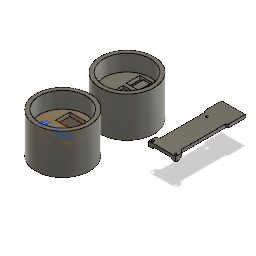
tstick_cap v71(Fusion360) (Autodesk Fusion 360 design; units mm, degrees)
Autodesk Fusion 360 part; units mm, degrees
sketch "Sketch1" plane through (0, 0, 0) normal (0, 1, 0) x (1, 0, 0) in component "battery_cap"
  circle A0 centre (0, 0) radius 21.25
  circle A1 centre (0, 0) radius 24.75
  dimension "d29" = 42.5
  dimension "d30" = 3.5
  constraint coincident A0.centre A1.centre
  measures "d29" diameter of A0
extrude "Extrude4" add sketch "Sketch1" against normal blind 3.5 contours A0 | A1 makes body 1 in component "battery_cap"
extrude "Extrude5" add sketch "Sketch1" along normal blind 15 bodies 1 in component "battery_cap"
sketch "Sketch2" plane through (0, -3.5, 0) normal (0, -1, 0) x (1, 0, 0) in component "battery_cap"
  circle A0 centre (0, 0) radius 24.75
  circle A1 centre (0, 0) radius 21.25
extrude "Extrude6" add sketch "Sketch2" along normal blind 15 bodies 1 in component "battery_cap"
sketch "switch_battery" plane through (0, -3.5, 0) normal (0, -1, 0) x (1, 0, 0) in component "battery_cap"
  circle A0 centre (0, 0) radius 21.25
  line L0 (0, 0) -> (0, 32) construction
  line L1 (0, 0) -> (28, 0) construction
  line L2 (28, 0) -> (27, 0)
  line L3 (9.5, -16) -> (-9.5, -16)
  line L4 (-9.5, -16) -> (-9.5, -3)
  line L5 (-9.5, -3) -> (9.5, -3)
  line L6 (9.5, -3) -> (9.5, -16)
  line L7 (9.5, -16) -> (-9.5, -3) construction
  line L8 (-9.5, -16) -> (9.5, -3) construction
  line L9 (11.725, 6.6) -> (-11.725, 6.6)
  line L10 (-11.725, 6.6) -> (-11.725, 1)
  line L11 (-11.725, 1) -> (11.725, 1)
  line L12 (11.725, 1) -> (11.725, 6.6)
  line L13 (11.725, 6.6) -> (-11.725, 1) construction
  line L14 (-11.725, 6.6) -> (11.725, 1) construction
  line L15 (11.725, 6.6) -> (11.725, 8.6)
  line L16 (-11.725, 6.6) -> (-11.725, 8.6)
  line L17 (-11.725, 8.6) -> (11.725, 8.6)
  line L18 (11.725, 1) -> (11.725, -1)
  line L19 (-11.725, 1) -> (-11.725, -1)
  line L20 (-11.725, -1) -> (11.725, -1)
  point P0 (0, -9.5)
  point P1 (0, 3.8)
  dimension "d48" = 19
  dimension "d49" = 13
  dimension "d50" = 3
  dimension "d51" = 23.45
  dimension "d52" = 5.6
  dimension "d53" = 1
  dimension "d181" = 2
  dimension "d182" = 2
  constraint coincident A0.centre L0.start
  constraint vertical L0
  constraint perpendicular L0 L1
  constraint coincident L1 L2.end
  constraint perpendicular L3 L4
  constraint parallel L3 L5
  constraint parallel L4 L6
  constraint horizontal L3
  constraint coincident L7 P0
  constraint coincident L8 P0
  constraint coincident L0 P0
  constraint perpendicular L9 L10
  constraint parallel L9 L11
  constraint parallel L10 L12
  constraint horizontal L9
  constraint coincident L13 P1
  constraint coincident L14 P1
  constraint coincident L0 P1
  constraint perpendicular L9 L15
  constraint perpendicular L9 L16
  constraint perpendicular L15 L17
  constraint perpendicular L1 L18
  constraint perpendicular L11 L19
  constraint perpendicular L18 L20
  measures "d48" distance of L4.end L5.end
  measures "d49" distance of L3.end L4.end
  measures "d50" distance of A0.centre L5
  measures "d51" distance of L10.end L11.end
  measures "d52" distance of L9.end L10.end
  measures "d53" distance of A0.centre L11
  measures "d181" distance of L9 L17
  measures "d182" distance of L11 L20
extrude "Extrude13" add sketch "switch_battery" along normal blind 15 contours L9 L15 L16 L17 | L11 L18 L19 L20 bodies 1 in component "battery_cap"
extrude "Extrude7" cut sketch "switch_battery" against normal up to surface (3.5 mm away) contours L3 L4 L5 L6 bodies 1 in component "battery_cap"
sketch "Sketch1 (2)" plane through (0, 0, 0) normal (0, 1, 0) x (1, 0, 0) in component "esp_cap"
  circle A0 centre (0, 0) radius 21.25
  circle A1 centre (0, 0) radius 24.75
  dimension "d29_1" = 42.5
  dimension "d30_1" = 3.5
  constraint coincident A0.centre A1.centre
  measures "d29_1" diameter of A0
extrude "Extrude4'" add sketch "Sketch1 (2)" against normal blind 3.5 separate body contours A0 | A1 makes body 2 in component "esp_cap"
extrude "Extrude5'" add sketch "Sketch1 (2)" along normal blind 15 bodies 2 in component "esp_cap"
sketch "Sketch2 (2)" plane through (0, -3.5, 0) normal (0, -1, 0) x (1, 0, 0) in component "esp_cap"
  circle A0 centre (0, 0) radius 24.75
  circle A1 centre (0, 0) radius 21.25
extrude "Extrude6'" add sketch "Sketch2 (2)" along normal blind 18.5 bodies 2 in component "esp_cap"
sketch "botton" plane through (0, -3.5, 0) normal (0, -1, 0) x (1, 0, 0) in component "esp_cap"
  circle A0 centre (0, 0) radius 21.25
  line L0 (0, 0) -> (0, 32) construction
  line L1 (0, 0) -> (30, 0) construction
  line L2 (-12.5, 6.5) -> (12.5, 6.5)
  line L3 (12.5, 6.5) -> (12.5, 5)
  line L4 (12.5, 5) -> (-12.5, 5)
  line L5 (-12.5, 5) -> (-12.5, 6.5)
  line L6 (-12.5, 6.5) -> (12.5, 5) construction
  line L7 (12.5, 6.5) -> (-12.5, 5) construction
  line L8 (7.4, 4.9) -> (12.4, 4.9)
  line L9 (12.4, 4.9) -> (12.4, -2.1)
  line L10 (12.4, -2.1) -> (7.4, -2.1)
  line L11 (7.4, -2.1) -> (7.4, 4.9)
  line L12 (7.4, 4.9) -> (12.4, -2.1) construction
  line L13 (12.4, 4.9) -> (7.4, -2.1) construction
  line L14 (-3.5, 4.9) -> (6.5, 4.9)
  line L15 (6.5, 4.9) -> (6.5, -0.1)
  line L16 (6.5, -0.1) -> (-3.5, -0.1)
  line L17 (-3.5, -0.1) -> (-3.5, 4.9)
  line L18 (-3.5, 4.9) -> (6.5, -0.1) construction
  line L19 (6.5, 4.9) -> (-3.5, -0.1) construction
  line L20 (0, 0) -> (0, -28) construction
  circle A1 centre (0, -12) radius 4
  line L21 (-6.25, -5.75) -> (6.25, -5.75)
  line L22 (6.25, -5.75) -> (6.25, -18.25)
  line L23 (6.25, -18.25) -> (-6.25, -18.25)
  line L24 (-6.25, -18.25) -> (-6.25, -5.75)
  line L25 (-6.25, -5.75) -> (6.25, -18.25) construction
  line L26 (6.25, -5.75) -> (-6.25, -18.25) construction
  line L27 (0, -12) -> (-10.4008, -12) construction
  line L28 (0, -12) -> (10, -12) construction
  line L29 (7.25, -13.5) -> (6.25, -13.5)
  line L30 (6.25, -13.5) -> (6.25, -10.5)
  line L31 (6.25, -10.5) -> (7.25, -10.5)
  line L32 (7.25, -10.5) -> (7.25, -13.5)
  line L33 (7.25, -13.5) -> (6.25, -10.5) construction
  line L34 (6.25, -13.5) -> (7.25, -10.5) construction
  line L35 (-7.25, -13.5) -> (-6.25, -13.5)
  line L36 (-6.25, -10.5) -> (-7.25, -10.5)
  line L37 (-7.25, -10.5) -> (-7.25, -13.5)
  line L38 (-6.25, -13.5) -> (-6.25, -10.5)
  line L39 (7.5, 5) -> (7.5, 6.5)
  line L40 (-7.5, 5) -> (-7.5, 6.5)
  line L41 (12.5, 6.5) -> (7.5, 6.5)
  line L42 (7.5, 9.75) -> (12.5, 9.75)
  line L43 (12.5, 9.75) -> (12.5, 6.5)
  line L44 (-12.5, 6.5) -> (-7.5, 6.5)
  line L45 (-7.1372, 9.75) -> (-12.5, 9.75)
  line L46 (-12.5, 9.75) -> (-12.5, 6.5)
  line L47 (12.5, 9.75) -> (-12.5, 9.75)
  line L48 (-12.5, 9.75) -> (-12.5, 11.25)
  line L49 (-12.5, 11.25) -> (12.5, 11.25)
  line L50 (12.5, 11.25) -> (12.5, 9.75)
  line L51 (11, 6.5) -> (11, 11.5)
  line L52 (-11, 6.5) -> (-11, 9.75)
  point P0 (0, 5.75)
  point P1 (9.9, 1.4)
  point P2 (1.5, 2.4)
  point P3 (0, -12)
  point P4 (6.75, -12)
  dimension "d65" = 25
  dimension "d66" = 1.5
  dimension "d67" = 5
  dimension "d70" = 5
  dimension "d71" = 7
  dimension "d72" = 0.1
  dimension "d74" = 10
  dimension "d75" = 5
  dimension "d76" = 0.1
  dimension "d82" = 0.1
  dimension "d83" = 9
  dimension "d111" = 8
  dimension "d112" = 12
  dimension "d113" = 12.5
  dimension "d114" = 12.5
  dimension "d117" = 1
  dimension "d118" = 3
  dimension "d119" = 6.25
  dimension "d200" = 5
  dimension "d201" = 5
  dimension "d202" = 3.25
  dimension "d203" = 3.25
  dimension "d204" = 1.5
  dimension "d205" = 1.5
  dimension "d206" = 1.5
  constraint coincident A0.centre L0.start
  constraint vertical L0
  constraint perpendicular L0 L1
  constraint perpendicular L2 L3
  constraint parallel L2 L4
  constraint parallel L3 L5
  constraint horizontal L2
  constraint coincident L6 P0
  constraint coincident L7 P0
  constraint coincident L0 P0
  constraint perpendicular L8 L9
  constraint parallel L8 L10
  constraint parallel L9 L11
  constraint horizontal L8
  constraint coincident L12 P1
  constraint coincident L13 P1
  constraint perpendicular L14 L15
  constraint parallel L14 L16
  constraint parallel L15 L17
  constraint horizontal L14
  constraint coincident L18 P2
  constraint coincident L19 P2
  constraint parallel L0 L20
  constraint coincident L20 P3
  constraint perpendicular L21 L22
  constraint parallel L21 L23
  constraint parallel L22 L24
  constraint horizontal L21
  constraint coincident L25 P3
  constraint coincident L26 P3
  constraint coincident P3 A1.centre
  constraint horizontal L27
  constraint perpendicular L20 L28
  constraint perpendicular L29 L30
  constraint parallel L29 L31
  constraint parallel L30 L32
  constraint horizontal L29
  constraint coincident L33 P4
  constraint coincident L34 P4
  constraint coincident L28 P4
  constraint symmetric L20 L29.start L35.start
  constraint symmetric L20 L29.end L35.end
  constraint symmetric L20 L30.end L36.start
  constraint symmetric L20 L31.end L36.end
  constraint coincident L4 L39.start
  constraint coincident L2 L39.end
  constraint perpendicular L2 L39
  constraint coincident L4 L40.start
  constraint coincident L2 L40.end
  constraint perpendicular L2 L40
  constraint parallel L41 L42
  constraint parallel L44 L45
  constraint perpendicular L47 L48
  constraint parallel L47 L49
  constraint parallel L48 L50
  constraint vertical L51
  constraint coincident L41 L51.start
  constraint coincident L2 L52.start
  constraint coincident L47 L52.end
  constraint perpendicular L47 L52
  measures "d65" distance of L3.end L4.end
  measures "d66" distance of L2.end L3.end
  measures "d67" distance of A0.centre L4
  measures "d70" distance of L9 L11
  measures "d71" distance of L8 L10
  measures "d72" distance of L4 L8
  measures "d74" distance of L15.end L16.end
  measures "d75" distance of L14.end L15.end
  measures "d76" distance of L4 L14
  measures "d82" distance of L3 L9
  measures "d83" distance of L5 L17
  measures "d111" diameter of A1
  measures "d112" distance of A0.centre P3
  measures "d113" distance of L22.end L23.end
  measures "d114" distance of L21.end L22.end
  measures "d117" distance of L30.end L31.end
  measures "d118" distance of L29 L31
  measures "d119" distance of P3 L30
  measures "d200" distance of L3 L39
  measures "d201" distance of L5 L40
  measures "d202" distance of L44 L45
  measures "d203" distance of L2 L42
  measures "d204" distance of L47 L49
  measures "d205" distance of L43 L51
  measures "d206" distance of L46 L52
extrude "Extrude30" add sketch "botton" along normal blind 18.5 contours L2 L44 L45 L46 L47 L52 | L2 L4 L5 L40 L44 | L42 L45 L47 L48 L49 L51 | L2 L3 L4 L39 L41 | L42 L47 L49 L50 L51 | L2 L41 L42 L43 L47 L51 bodies 2 in component "esp_cap"
extrude "Extrude11" cut sketch "botton" against normal up to surface (3.5 mm away) contours L8 L9 L10 L11 bodies 2 in component "esp_cap"
extrude "Extrude12" cut sketch "botton" against normal up to surface (3.5 mm away) contours L14 L15 L16 L17 bodies 2 in component "esp_cap"
sketch "top" plane through (0, 0, 0) normal (0, 1, 0) x (-1, 0, 0) in component "esp_cap"
  line L0 (3.5, 4.9) -> (3.5, -0.1)
  line L1 (3.5, -0.1) -> (-6.5, -0.1)
  line L2 (-6.5, 4.9) -> (3.5, 4.9)
  line L3 (-7.4, 4.9) -> (-7.4, -2.1)
  line L4 (-7.4, -2.1) -> (-12.4, -2.1)
  line L5 (-12.4, -2.1) -> (-12.4, 4.9)
  circle A0 centre (0, 0) radius 21.25
  line L6 (0, 0) -> (-32, 0) construction
  line L7 (0, 0) -> (0, -28) construction
  line L8 (-9, 7.4) -> (6, 7.4)
  line L9 (6, 7.4) -> (6, -2.6)
  line L10 (6, -2.6) -> (-9, -2.6)
  line L11 (-9, -2.6) -> (-9, 7.4)
  line L12 (-6.5, -0.1) -> (-6.5, 4.9)
  line L13 (-12.4, 4.9) -> (-7.4, 4.9)
  line L14 (0, 0) -> (27, 0) construction
  line L15 (-6, -5.7474) -> (6.5, -5.7474)
  line L16 (6.5, -5.7474) -> (6.5, -18.2474)
  line L17 (6.5, -18.2474) -> (-6, -18.2474)
  line L18 (-6, -18.2474) -> (-6, -5.7474)
  line L19 (-6, -5.7474) -> (6.5, -18.2474) construction
  line L20 (6.5, -5.7474) -> (-6, -18.2474) construction
  line L21 (3.375, -18.2474) -> (-2.875, -18.2474)
  line L22 (-2.875, -18.2474) -> (-2.875, -5.7474)
  line L23 (-2.875, -5.7474) -> (3.375, -5.7474)
  line L24 (3.375, -5.7474) -> (3.375, -18.2474)
  line L25 (3.375, -18.2474) -> (-2.875, -5.7474) construction
  line L26 (-2.875, -18.2474) -> (3.375, -5.7474) construction
  line L27 (10.5318, 13.8673) -> (10.5318, 8.8166)
  line L28 (10.5318, 8.8166) -> (12.4185, 8.8166)
  line L29 (12.4185, 8.8166) -> (12.4185, 8.1408)
  line L30 (12.4185, 8.1408) -> (7.8794, 8.1408)
  line L31 (7.8794, 8.1408) -> (7.8794, 8.8166)
  line L32 (7.8794, 8.8166) -> (9.7739, 8.8166)
  line L33 (9.7739, 8.8166) -> (9.7739, 13.8673)
  line L34 (9.7739, 13.8673) -> (10.5318, 13.8673)
  line L35 (7.4653, 12.1486) -> (7.4653, 11.4416)
  line L36 (7.4653, 11.4416) -> (5.3052, 11.4416)
  line L37 (5.3052, 11.4416) -> (5.3052, 12.1486)
  line L38 (5.3052, 12.1486) -> (7.4653, 12.1486)
  line L39 (4.6958, 12.0275) -> (3.981, 11.965)
  spline S0 degree 3 poles (3.981, 11.965) (3.9608, 12.0982) (3.9232, 12.3477) (3.8027, 12.5689) (3.7466, 12.672) knots 0 0 0 0 0.040051 0.074995 0.074995 0.074995 0.074995
  spline S1 degree 3 poles (3.7466, 12.672) (3.6718, 12.7606) (3.5115, 12.9503) (3.2878, 13.0592) (3.1685, 13.1173) knots 0 0 0 0 0.034396 0.07369 0.07369 0.07369 0.07369
  spline S2 degree 3 poles (3.1685, 13.1173) (3.0315, 13.1663) (2.7474, 13.2679) (2.4458, 13.2794) (2.2896, 13.2853) knots 0 0 0 0 0.043374 0.08995 0.08995 0.08995 0.08995
  spline S3 degree 3 poles (2.2896, 13.2853) (2.1524, 13.2811) (1.8911, 13.2731) (1.6422, 13.194) (1.5239, 13.1564) knots 0 0 0 0 0.040947 0.077974 0.077974 0.077974 0.077974
  spline S4 degree 3 poles (1.5239, 13.1564) (1.4226, 13.1124) (1.2331, 13.0302) (1.0957, 12.8764) (1.0318, 12.8048) knots 0 0 0 0 0.032675 0.061126 0.061126 0.061126 0.061126
  spline S5 degree 3 poles (1.0318, 12.8048) (0.9839, 12.7283) (0.8895, 12.5774) (0.8749, 12.4001) (0.8677, 12.3127) knots 0 0 0 0 0.026644 0.052557 0.052557 0.052557 0.052557
  spline S6 degree 3 poles (0.8677, 12.3127) (0.8737, 12.2263) (0.8857, 12.0566) (0.9784, 11.914) (1.0239, 11.8439) knots 0 0 0 0 0.025496 0.050141 0.050141 0.050141 0.050141
  spline S7 degree 3 poles (1.0239, 11.8439) (1.0898, 11.7771) (1.237, 11.6276) (1.4319, 11.548) (1.5396, 11.5041) knots 0 0 0 0 0.027866 0.062324 0.062324 0.062324 0.062324
  spline S8 degree 3 poles (1.5396, 11.5041) (1.6626, 11.4648) (1.9983, 11.3575) (2.3416, 11.2774) (2.5591, 11.2267) knots 0 0 0 0 0.038735 0.105693 0.105693 0.105693 0.105693
  spline S9 degree 3 poles (2.5591, 11.2267) (2.7852, 11.1721) (3.1633, 11.0809) (3.5208, 10.9286) (3.6646, 10.8673) knots 0 0 0 0 0.069608 0.116413 0.116413 0.116413 0.116413
  spline S10 degree 3 poles (3.6646, 10.8673) (3.7905, 10.7947) (4.0295, 10.6569) (4.1981, 10.4391) (4.2778, 10.3361) knots 0 0 0 0 0.043147 0.081832 0.081832 0.081832 0.081832
  spline S11 degree 3 poles (4.2778, 10.3361) (4.336, 10.2255) (4.4536, 10.0015) (4.4692, 9.749) (4.4771, 9.6212) knots 0 0 0 0 0.037035 0.074961 0.074961 0.074961 0.074961
  spline S12 degree 3 poles (4.4771, 9.6212) (4.4664, 9.4786) (4.445, 9.1907) (4.3027, 8.9394) (4.231, 8.8127) knots 0 0 0 0 0.042344 0.085459 0.085459 0.085459 0.085459
  spline S13 degree 3 poles (4.231, 8.8127) (4.137, 8.693) (3.9427, 8.4455) (3.6589, 8.309) (3.5122, 8.2384) knots 0 0 0 0 0.045005 0.093093 0.093093 0.093093 0.093093
  spline S14 degree 3 poles (3.5122, 8.2384) (3.3474, 8.1815) (3.0071, 8.0639) (2.6471, 8.0502) (2.4614, 8.0431) knots 0 0 0 0 0.052008 0.107399 0.107399 0.107399 0.107399
  spline S15 degree 3 poles (2.4614, 8.0431) (2.2599, 8.0499) (1.8756, 8.0629) (1.5129, 8.1898) (1.3403, 8.2502) knots 0 0 0 0 0.060087 0.114591 0.114591 0.114591 0.114591
  spline S16 degree 3 poles (1.3403, 8.2502) (1.1883, 8.3241) (0.8925, 8.4679) (0.6892, 8.7262) (0.5903, 8.8517) knots 0 0 0 0 0.049979 0.097264 0.097264 0.097264 0.097264
  spline S17 degree 3 poles (0.5903, 8.8517) (0.5132, 8.9901) (0.3564, 9.2712) (0.325, 9.5915) (0.3091, 9.7541) knots 0 0 0 0 0.047003 0.095424 0.095424 0.095424 0.095424
  line L40 (0.3091, 9.7541) -> (1.0357, 9.8087)
  spline S18 degree 3 poles (1.0357, 9.8087) (1.0631, 9.6421) (1.1148, 9.328) (1.3321, 9.0969) (1.4341, 8.9884) knots 0 0 0 0 0.049369 0.093051 0.093051 0.093051 0.093051
  spline S19 degree 3 poles (1.4341, 8.9884) (1.5697, 8.9078) (1.8751, 8.7263) (2.2319, 8.7165) (2.4302, 8.7111) knots 0 0 0 0 0.046599 0.104923 0.104923 0.104923 0.104923
  spline S20 degree 3 poles (2.4302, 8.7111) (2.6334, 8.7143) (2.99, 8.72) (3.3005, 8.8913) (3.4341, 8.965) knots 0 0 0 0 0.05981 0.104943 0.104943 0.104943 0.104943
  spline S21 degree 3 poles (3.4341, 8.965) (3.5252, 9.0506) (3.7014, 9.216) (3.7319, 9.455) (3.7466, 9.5705) knots 0 0 0 0 0.036237 0.070062 0.070062 0.070062 0.070062
  spline S22 degree 3 poles (3.7466, 9.5705) (3.7377, 9.6685) (3.72, 9.8627) (3.5889, 10.0069) (3.5239, 10.0783) knots 0 0 0 0 0.028671 0.056816 0.056816 0.056816 0.056816
  spline S23 degree 3 poles (3.5239, 10.0783) (3.3944, 10.1507) (3.0385, 10.3497) (2.638, 10.4345) (2.3833, 10.4884) knots 0 0 0 0 0.04433 0.121785 0.121785 0.121785 0.121785
  spline S24 degree 3 poles (2.3833, 10.4884) (2.1212, 10.5463) (1.6903, 10.6414) (1.276, 10.7925) (1.1138, 10.8517) knots 0 0 0 0 0.080411 0.132172 0.132172 0.132172 0.132172
  spline S25 degree 3 poles (1.1138, 10.8517) (0.9611, 10.9293) (0.6748, 11.0749) (0.4708, 11.3222) (0.3755, 11.4377) knots 0 0 0 0 0.050729 0.095154 0.095154 0.095154 0.095154
  spline S26 degree 3 poles (0.3755, 11.4377) (0.306, 11.561) (0.1639, 11.8132) (0.1463, 12.1024) (0.1372, 12.2502) knots 0 0 0 0 0.041894 0.08566 0.08566 0.08566 0.08566
  spline S27 degree 3 poles (0.1372, 12.2502) (0.1488, 12.4014) (0.1722, 12.7083) (0.3226, 12.9771) (0.3989, 13.1134) knots 0 0 0 0 0.044913 0.091178 0.091178 0.091178 0.091178
  spline S28 degree 3 poles (0.3989, 13.1134) (0.4983, 13.2414) (0.7035, 13.5057) (0.9999, 13.6618) (1.1528, 13.7423) knots 0 0 0 0 0.048003 0.099191 0.099191 0.099191 0.099191
  spline S29 degree 3 poles (1.1528, 13.7423) (1.3241, 13.8073) (1.6789, 13.9417) (2.0582, 13.9571) (2.2544, 13.965) knots 0 0 0 0 0.054571 0.11304 0.11304 0.11304 0.11304
  spline S30 degree 3 poles (2.2544, 13.965) (2.495, 13.9589) (2.9416, 13.9475) (3.3642, 13.8044) (3.5591, 13.7384) knots 0 0 0 0 0.071708 0.133092 0.133092 0.133092 0.133092
  spline S31 degree 3 poles (3.5591, 13.7384) (3.7236, 13.6545) (4.0486, 13.4886) (4.2727, 13.2008) (4.3833, 13.0587) knots 0 0 0 0 0.054682 0.107998 0.107998 0.107998 0.107998
  spline S32 degree 3 poles (4.3833, 13.0587) (4.4706, 12.9002) (4.6476, 12.5787) (4.6796, 12.2129) (4.6958, 12.0275) knots 0 0 0 0 0.053651 0.108817 0.108817 0.108817 0.108817
  line L41 (-2.3432, 13.2384) -> (-2.4448, 13.8595)
  spline S33 degree 3 poles (-2.4448, 13.8595) (-2.3514, 13.8777) (-2.1758, 13.9119) (-1.9971, 13.9188) (-1.9136, 13.922) knots 0 0 0 0 0.028513 0.053562 0.053562 0.053562 0.053562
  spline S34 degree 3 poles (-1.9136, 13.922) (-1.7985, 13.9198) (-1.5926, 13.9159) (-1.4034, 13.8361) (-1.3198, 13.8009) knots 0 0 0 0 0.034119 0.061085 0.061085 0.061085 0.061085
  spline S35 degree 3 poles (-1.3198, 13.8009) (-1.2553, 13.7587) (-1.1306, 13.6771) (-1.058, 13.5472) (-1.0229, 13.4845) knots 0 0 0 0 0.022757 0.043965 0.043965 0.043965 0.043965
  spline S36 degree 3 poles (-1.0229, 13.4845) (-0.9982, 13.3824) (-0.9323, 13.1097) (-0.9352, 12.8284) (-0.937, 12.6525) knots 0 0 0 0 0.03143 0.083915 0.083915 0.083915 0.083915
  line L42 (-0.937, 12.6525) -> (-0.937, 10.2658)
  line L43 (-0.937, 10.2658) -> (-0.4214, 10.2658)
  line L44 (-0.4214, 10.2658) -> (-0.4214, 9.7189)
  line L45 (-0.4214, 9.7189) -> (-0.937, 9.7189)
  line L46 (-0.937, 9.7189) -> (-0.937, 8.6916)
  line L47 (-0.937, 8.6916) -> (-1.6362, 8.2697)
  line L48 (-1.6362, 8.2697) -> (-1.6362, 9.7189)
  line L49 (-1.6362, 9.7189) -> (-2.3432, 9.7189)
  line L50 (-2.3432, 9.7189) -> (-2.3432, 10.2658)
  line L51 (-2.3432, 10.2658) -> (-1.6362, 10.2658)
  line L52 (-1.6362, 10.2658) -> (-1.6362, 12.6916)
  spline S37 degree 3 poles (-1.6362, 12.6916) (-1.6352, 12.7744) (-1.6337, 12.9047) (-1.6613, 13.0319) (-1.6714, 13.0783) knots 0 0 0 0 0.024723 0.038934 0.038934 0.038934 0.038934
  spline S38 degree 3 poles (-1.6714, 13.0783) (-1.6863, 13.1055) (-1.7162, 13.1603) (-1.7669, 13.1967) (-1.7925, 13.215) knots 0 0 0 0 0.009183 0.018473 0.018473 0.018473 0.018473
  spline S39 degree 3 poles (-1.7925, 13.215) (-1.8265, 13.2298) (-1.9035, 13.2632) (-1.9877, 13.2648) (-2.0347, 13.2658) knots 0 0 0 0 0.01103 0.024955 0.024955 0.024955 0.024955
  spline S40 degree 3 poles (-2.0347, 13.2658) (-2.08, 13.2642) (-2.1833, 13.2605) (-2.2857, 13.2464) (-2.3432, 13.2384) knots 0 0 0 0 0.013591 0.030998 0.030998 0.030998 0.030998
  line L53 (-3.0347, 8.9494) -> (-3.0347, 8.1408)
  line L54 (-3.0347, 8.1408) -> (-3.7378, 8.1408)
  line L55 (-3.7378, 8.1408) -> (-3.7378, 8.9494)
  line L56 (-3.7378, 8.9494) -> (-3.0347, 8.9494)
  line L57 (-3.0347, 13.8673) -> (-3.0347, 9.7189)
  line L58 (-3.0347, 9.7189) -> (-3.7378, 9.7189)
  line L59 (-3.7378, 9.7189) -> (-3.7378, 13.8673)
  line L60 (-3.7378, 13.8673) -> (-3.0347, 13.8673)
  line L61 (-7.5151, 12.3478) -> (-8.2065, 12.4377)
  spline S41 degree 3 poles (-8.2065, 12.4377) (-8.1575, 12.6599) (-8.0634, 13.0865) (-7.7666, 13.4058) (-7.6245, 13.5588) knots 0 0 0 0 0.066897 0.128377 0.128377 0.128377 0.128377
  spline S42 degree 3 poles (-7.6245, 13.5588) (-7.4576, 13.6761) (-7.1144, 13.9174) (-6.6953, 13.9463) (-6.48, 13.9611) knots 0 0 0 0 0.059996 0.123397 0.123397 0.123397 0.123397
  spline S43 degree 3 poles (-6.48, 13.9611) (-6.2129, 13.9411) (-5.6956, 13.9024) (-5.3002, 13.5681) (-5.1089, 13.4064) knots 0 0 0 0 0.078096 0.151317 0.151317 0.151317 0.151317
  spline S44 degree 3 poles (-5.1089, 13.4064) (-4.9588, 13.1874) (-4.6304, 12.7082) (-4.6063, 12.1253) (-4.5932, 11.8087) knots 0 0 0 0 0.078115 0.17091 0.17091 0.17091 0.17091
  spline S45 degree 3 poles (-4.5932, 11.8087) (-4.6005, 11.5966) (-4.6142, 11.1929) (-4.751, 10.8131) (-4.8159, 10.633) knots 0 0 0 0 0.063234 0.120321 0.120321 0.120321 0.120321
  spline S46 degree 3 poles (-4.8159, 10.633) (-4.8984, 10.4763) (-5.0607, 10.1682) (-5.3496, 9.9744) (-5.4917, 9.8791) knots 0 0 0 0 0.052205 0.102672 0.102672 0.102672 0.102672
  spline S47 degree 3 poles (-5.4917, 9.8791) (-5.6478, 9.805) (-5.962, 9.656) (-6.3092, 9.6355) (-6.4839, 9.6252) knots 0 0 0 0 0.05132 0.103272 0.103272 0.103272 0.103272
  spline S48 degree 3 poles (-6.4839, 9.6252) (-6.6943, 9.636) (-7.0931, 9.6566) (-7.4302, 9.8687) (-7.5893, 9.9689) knots 0 0 0 0 0.062024 0.1175 0.1175 0.1175 0.1175
  spline S49 degree 3 poles (-7.5893, 9.9689) (-7.7205, 10.0984) (-7.9944, 10.369) (-8.0902, 10.7428) (-8.1401, 10.9377) knots 0 0 0 0 0.054233 0.113322 0.113322 0.113322 0.113322
  line L62 (-8.1401, 10.9377) -> (-7.4565, 11.0431)
  spline S50 degree 3 poles (-7.4565, 11.0431) (-7.4211, 10.9155) (-7.355, 10.6776) (-7.1868, 10.4976) (-7.1089, 10.4142) knots 0 0 0 0 0.039056 0.072807 0.072807 0.072807 0.072807
  spline S51 degree 3 poles (-7.1089, 10.4142) (-7.0212, 10.3527) (-6.8418, 10.2269) (-6.623, 10.2113) (-6.5112, 10.2033) knots 0 0 0 0 0.031506 0.06445 0.06445 0.06445 0.06445
  spline S52 degree 3 poles (-6.5112, 10.2033) (-6.3432, 10.2183) (-6.0117, 10.2481) (-5.7681, 10.4744) (-5.6479, 10.5861) knots 0 0 0 0 0.049087 0.09686 0.09686 0.09686 0.09686
  spline S53 degree 3 poles (-5.6479, 10.5861) (-5.5515, 10.7455) (-5.3293, 11.1128) (-5.3207, 11.5447) (-5.3159, 11.7892) knots 0 0 0 0 0.054986 0.126756 0.126756 0.126756 0.126756
  spline S54 degree 3 poles (-5.3159, 11.7892) (-5.32, 12.0363) (-5.3272, 12.4701) (-5.5432, 12.8434) (-5.6362, 13.0041) knots 0 0 0 0 0.072611 0.127467 0.127467 0.127467 0.127467
  spline S55 degree 3 poles (-5.6362, 13.0041) (-5.7521, 13.1146) (-5.9863, 13.3381) (-6.309, 13.3679) (-6.4722, 13.383) knots 0 0 0 0 0.046586 0.094217 0.094217 0.094217 0.094217
  spline S56 degree 3 poles (-6.4722, 13.383) (-6.6032, 13.3736) (-6.8584, 13.3552) (-7.0637, 13.2031) (-7.1636, 13.1291) knots 0 0 0 0 0.038515 0.075027 0.075027 0.075027 0.075027
  spline S57 degree 3 poles (-7.1636, 13.1291) (-7.2484, 13.026) (-7.4356, 12.7985) (-7.487, 12.5072) (-7.5151, 12.3478) knots 0 0 0 0 0.039394 0.086964 0.086964 0.086964 0.086964
  line L63 (-8.812, 13.8673) -> (-8.812, 8.1408)
  line L64 (-8.812, 8.1408) -> (-9.5151, 8.1408)
  line L65 (-9.5151, 8.1408) -> (-9.5151, 11.4064)
  line L66 (-9.5151, 11.4064) -> (-11.1792, 9.7189)
  line L67 (-11.1792, 9.7189) -> (-12.0893, 9.7189)
  line L68 (-12.0893, 9.7189) -> (-10.5034, 11.258)
  line L69 (-10.5034, 11.258) -> (-12.2495, 13.8673)
  line L70 (-12.2495, 13.8673) -> (-11.3823, 13.8673)
  line L71 (-11.3823, 13.8673) -> (-10.0112, 11.7462)
  line L72 (-10.0112, 11.7462) -> (-9.5151, 12.2228)
  line L73 (-9.5151, 12.2228) -> (-9.5151, 13.8673)
  line L74 (-9.5151, 13.8673) -> (-8.812, 13.8673)
  line L75 (7.6067, 18.9989) -> (7.6067, 14.704)
  line L76 (7.6067, 14.704) -> (7.0383, 14.704)
  line L77 (7.0383, 14.704) -> (7.0383, 18.9989)
  line L78 (7.0383, 18.9989) -> (7.6067, 18.9989)
  line L79 (6.0363, 18.9989) -> (6.0363, 14.704)
  line L80 (6.0363, 14.704) -> (4.5568, 14.704)
  spline S58 degree 3 poles (4.5568, 14.704) (4.4092, 14.7046) (4.1526, 14.7056) (3.8996, 14.7477) (3.7922, 14.7655) knots 0 0 0 0 0.044192 0.07682 0.07682 0.07682 0.07682
  spline S59 degree 3 poles (3.7922, 14.7655) (3.6749, 14.7985) (3.4461, 14.863) (3.2553, 15.0043) (3.1623, 15.0731) knots 0 0 0 0 0.036228 0.07062 0.07062 0.07062 0.07062
  spline S60 degree 3 poles (3.1623, 15.0731) (3.0557, 15.1769) (2.8384, 15.3885) (2.7172, 15.6667) (2.6555, 15.8085) knots 0 0 0 0 0.044179 0.090072 0.090072 0.090072 0.090072
  spline S61 degree 3 poles (2.6555, 15.8085) (2.6059, 15.9664) (2.5019, 16.2982) (2.4912, 16.6459) (2.4856, 16.828) knots 0 0 0 0 0.049425 0.103791 0.103791 0.103791 0.103791
  spline S62 degree 3 poles (2.4856, 16.828) (2.4892, 16.9826) (2.4961, 17.2759) (2.5665, 17.5606) (2.5998, 17.6952) knots 0 0 0 0 0.046231 0.087702 0.087702 0.087702 0.087702
  spline S63 degree 3 poles (2.5998, 17.6952) (2.6384, 17.8127) (2.711, 18.0336) (2.8348, 18.2302) (2.8928, 18.3221) knots 0 0 0 0 0.036947 0.069434 0.069434 0.069434 0.069434
  spline S64 degree 3 poles (2.8928, 18.3221) (2.9522, 18.3988) (3.0661, 18.5458) (3.2144, 18.658) (3.2854, 18.7118) knots 0 0 0 0 0.028941 0.055527 0.055527 0.055527 0.055527
  spline S65 degree 3 poles (3.2854, 18.7118) (3.3618, 18.7564) (3.5231, 18.8505) (3.7033, 18.8998) (3.7981, 18.9257) knots 0 0 0 0 0.026441 0.055764 0.055764 0.055764 0.055764
  spline S66 degree 3 poles (3.7981, 18.9257) (3.9049, 18.947) (4.1321, 18.9924) (4.3638, 18.9966) (4.4865, 18.9989) knots 0 0 0 0 0.032619 0.069359 0.069359 0.069359 0.069359
  line L81 (4.4865, 18.9989) -> (6.0363, 18.9989)
  line L82 (5.468, 18.4921) -> (4.551, 18.4921)
  spline S67 degree 3 poles (4.551, 18.4921) (4.4241, 18.4908) (4.1993, 18.4887) (3.981, 18.4359) (3.8859, 18.413) knots 0 0 0 0 0.037918 0.067164 0.067164 0.067164 0.067164
  spline S68 degree 3 poles (3.8859, 18.413) (3.8107, 18.3855) (3.6687, 18.3337) (3.5534, 18.2361) (3.4992, 18.1903) knots 0 0 0 0 0.023813 0.044936 0.044936 0.044936 0.044936
  spline S69 degree 3 poles (3.4992, 18.1903) (3.4347, 18.1142) (3.2977, 17.9527) (3.2245, 17.7536) (3.1858, 17.6483) knots 0 0 0 0 0.029693 0.063046 0.063046 0.063046 0.063046
  spline S70 degree 3 poles (3.1858, 17.6483) (3.1525, 17.5228) (3.0805, 17.2513) (3.0746, 16.9703) (3.0715, 16.8192) knots 0 0 0 0 0.038824 0.083958 0.083958 0.083958 0.083958
  spline S71 degree 3 poles (3.0715, 16.8192) (3.0754, 16.6173) (3.0823, 16.2569) (3.2294, 15.9292) (3.2942, 15.785) knots 0 0 0 0 0.059806 0.106748 0.106748 0.106748 0.106748
  spline S72 degree 3 poles (3.2942, 15.785) (3.3679, 15.6754) (3.5069, 15.4687) (3.7269, 15.353) (3.8303, 15.2987) knots 0 0 0 0 0.038914 0.0734 0.0734 0.0734 0.0734
  spline S73 degree 3 poles (3.8303, 15.2987) (3.9292, 15.2733) (4.1699, 15.2113) (4.4189, 15.211) (4.5656, 15.2108) knots 0 0 0 0 0.03053 0.07431 0.07431 0.07431 0.07431
  line L83 (4.5656, 15.2108) -> (5.468, 15.2108)
  line L84 (5.468, 15.2108) -> (5.468, 18.4921)
  line L85 (1.7209, 18.9989) -> (1.7209, 14.704)
  line L86 (1.7209, 14.704) -> (0.8654, 14.704)
  line L87 (0.8654, 14.704) -> (-0.1512, 17.745)
  spline S74 degree 3 poles (-0.1512, 17.745) (-0.1921, 17.8686) (-0.262, 18.0801) (-0.3286, 18.2925) (-0.3562, 18.3807) knots 0 0 0 0 0.039074 0.066801 0.066801 0.066801 0.066801
  spline S75 degree 3 poles (-0.3562, 18.3807) (-0.3872, 18.2842) (-0.4612, 18.054) (-0.5394, 17.8252) (-0.5848, 17.6923) knots 0 0 0 0 0.030412 0.072542 0.072542 0.072542 0.072542
  line L88 (-0.5848, 17.6923) -> (-1.6131, 14.704)
  line L89 (-1.6131, 14.704) -> (-2.3777, 14.704)
  line L90 (-2.3777, 14.704) -> (-2.3777, 18.9989)
  line L91 (-2.3777, 18.9989) -> (-1.8299, 18.9989)
  line L92 (-1.8299, 18.9989) -> (-1.8299, 15.4042)
  line L93 (-1.8299, 15.4042) -> (-0.5818, 18.9989)
  line L94 (-0.5818, 18.9989) -> (-0.0691, 18.9989)
  line L95 (-0.0691, 18.9989) -> (1.1731, 15.3426)
  line L96 (1.1731, 15.3426) -> (1.1731, 18.9989)
  line L97 (1.1731, 18.9989) -> (1.7209, 18.9989)
  line L98 (-3.3914, 18.9989) -> (-3.3914, 14.704)
  line L99 (-3.3914, 14.704) -> (-3.9598, 14.704)
  line L100 (-3.9598, 14.704) -> (-3.9598, 18.9989)
  line L101 (-3.9598, 18.9989) -> (-3.3914, 18.9989)
  line L102 (-4.9383, 18.9989) -> (-4.9383, 14.704)
  line L103 (-4.9383, 14.704) -> (-5.5066, 14.704)
  line L104 (-5.5066, 14.704) -> (-5.5066, 18.4921)
  line L105 (-5.5066, 18.4921) -> (-7.6219, 18.4921)
  line L106 (-7.6219, 18.4921) -> (-7.6219, 18.9989)
  line L107 (-7.6219, 18.9989) -> (-4.9383, 18.9989)
  point P0 (0.25, -11.9974)
  point P1 (0.25, -11.9974)
  point P2 (0.25, -11.9974)
  dimension "d149" = 2.5
  dimension "d150" = 2.5
  dimension "d151" = 2.5
  dimension "d153" = 2.5
  dimension "d155" = 12.5
  dimension "d156" = 12.5
  dimension "d158" = 12
  dimension "d159" = 6.25
  dimension "d160" = 12.5
  constraint coincident A0.centre L6.start
  constraint parallel L1 L6
  constraint perpendicular L6 L7
  constraint parallel L2 L8
  constraint parallel L0 L9
  constraint parallel L1 L10
  constraint perpendicular L9 L14
  constraint perpendicular L15 L16
  constraint parallel L15 L17
  constraint parallel L16 L18
  constraint horizontal L15
  constraint coincident L19 P2
  constraint coincident L20 P2
  constraint coincident P2 P1
  constraint perpendicular L21 L22
  constraint parallel L21 L23
  constraint parallel L22 L24
  constraint horizontal L21
  constraint coincident L25 P2
  constraint coincident L26 P2
  measures "d149" distance of L0 L9
  measures "d150" distance of L2 L8
  measures "d151" distance of L1 L10
  measures "d153" distance of L11 L12
  measures "d155" distance of L16.end L17.end
  measures "d156" distance of L15.end L16.end
  measures "d158" distance of A0.centre P2
  measures "d159" distance of L22.end L23.end
  measures "d160" distance of L21.end L22.end
extrude "Extrude14" cut sketch "top" against normal blind 1 contours L75 L76 L77 L78 | L79 L80 S58 S59 S60 S61 S62 S63 S64 S65 S66 L81 | L85 L86 L87 S74 S75 L88 L89 L90 L91 L92 L93 L94 L95 L96 L97 | L98 L99 L100 L101 | L102 L103 L104 L105 L106 L107 bodies 1 in component "battery_cap"
extrude "Extrude31" cut sketch "top" against normal blind 1 contours L75 L76 L77 L78 | L79 L80 S58 S59 S60 S61 S62 S63 S64 S65 S66 L81 | L85 L86 L87 S74 S75 L88 L89 L90 L91 L92 L93 L94 L95 L96 L97 | L98 L99 L100 L101 | L102 L103 L104 L105 L106 L107 bodies 2 in component "esp_cap"
extrude "Extrude27" add sketch "top" along normal blind 1 contours L27 L28 L29 L30 L31 L32 L33 L34 | L35 L36 L37 L38 | L39 S0 S1 S2 S3 S4 S5 S6 S7 S8 S9 S10 S11 S12 S13 S14 S15 S16 S17 L40 S18 S19 S20 S21 S22 S23 S24 S25 S26 S27 S28 S29 S30 S31 S32 | L41 S33 S34 S35 S36 L42 L43 L44 L45 L46 L47 L48 L49 L50 L51 L52 S37 S38 S39 S40 | L53 L54 L55 L56 | L57 L58 L59 L60 | L61 S41 S42 S43 S44 S45 S46 S47 S48 S49 L62 S50 S51 S52 S53 S54 S55 S56 S57 | L63 L64 L65 L66 L67 L68 L69 L70 L71 L72 L73 L74 bodies 2 in component "esp_cap"
extrude "Extrude17" cut sketch "top" against normal blind 2.5 contours L3 L4 L8 L9 L10 L11 L13 | L3 L4 L11 L13 bodies 2 in component "esp_cap"
extrude "Extrude24" cut sketch "top" against normal blind 2 contours L15 L17 L21 L22 L23 L24 bodies 2 in component "esp_cap"
extrude "Extrude25" cut sketch "top" against normal up to surface (3.5 mm away) contours L15 L17 L18 L22 | L15 L16 L17 L24 bodies 2 in component "esp_cap"
extrude "Extrude26" add 1 faces at (9, -0.8333, -2.4333) along direction (-1, 0, 0) up to surface (1.6 mm away) on bodies 2 bodies 2 in component "esp_cap"
move_face "OffsetFaces1" offset 3.5 1 faces at (23.4121, -18.5, -2.2853) on bodies 1 in component "battery_cap"
sketch "top (2)" plane through (0, 0, 0) normal (0, 1, 0) x (-1, 0, 0) in component "battery_cap"
  circle A0 centre (0, 0) radius 21.25
  line L0 (-9.5, -16) -> (-9.5, -3)
  line L1 (-9.5, -3) -> (9.5, -3)
  line L2 (9.5, -3) -> (9.5, -16)
  line L3 (9.5, -16) -> (-9.5, -16)
sketch "bed" plane through (0, 0, 0) normal (0, 1, 0) x (1, 0, 0) in component "esp_bed"
  line L0 (12.5, 32.75) -> (-12.5, 32.75)
  line L1 (-12.5, 32.75) -> (-12.5, -32.75)
  line L2 (-12.5, -32.75) -> (12.5, -32.75)
  line L3 (12.5, -32.75) -> (12.5, 32.75)
  line L4 (12.5, 32.75) -> (-12.5, -32.75) construction
  line L5 (-12.5, 32.75) -> (12.5, -32.75) construction
  circle A0 centre (10.5, -30.75) radius 1
  circle A1 centre (-10.5, -30.75) radius 1
  circle A2 centre (-5, 13.25) radius 1
  line L6 (10.5, -30.75) -> (10.5, 25) construction
  line L7 (-19, 17.75) -> (17, 17.75) construction
  line L8 (-12.5, 17.75) -> (-9.4847, 16.0091)
  line L9 (-9.4847, 16.0091) -> (-9.4847, -24.85)
  line L10 (-9.4847, -24.85) -> (-12.5, -27.3801)
  line L11 (-12.5, -27.3801) -> (-12.5, 17.75)
  line L12 (0, -32.75) -> (0, 40) construction
  line L13 (12.5, -27.3801) -> (12.5, 17.75)
  line L14 (9.4847, 16.0091) -> (9.4847, -24.85)
  line L15 (12.5, 17.75) -> (9.4847, 16.0091)
  line L16 (9.4847, -24.85) -> (12.5, -27.3801)
  line L17 (8.5, -28.75) -> (12.5, -28.75)
  line L18 (12.5, -28.75) -> (12.5, -32.75)
  line L19 (12.5, -32.75) -> (8.5, -32.75)
  line L20 (8.5, -32.75) -> (8.5, -28.75)
  line L21 (8.5, -28.75) -> (12.5, -32.75) construction
  line L22 (12.5, -28.75) -> (8.5, -32.75) construction
  line L23 (-8.5, -28.75) -> (-12.5, -28.75)
  line L24 (-12.5, -28.75) -> (-12.5, -32.75)
  line L25 (-12.5, -32.75) -> (-8.5, -32.75)
  line L26 (-8.5, -32.75) -> (-8.5, -28.75)
  line L27 (-8.5, -28.75) -> (-12.5, -32.75) construction
  line L28 (-12.5, -28.75) -> (-8.5, -32.75) construction
  line L29 (-3, 11.25) -> (-7, 11.25)
  line L30 (-7, 11.25) -> (-7, 15.25)
  line L31 (-7, 15.25) -> (-3, 15.25)
  line L32 (-3, 15.25) -> (-3, 11.25)
  line L33 (-3, 11.25) -> (-7, 15.25) construction
  line L34 (-7, 11.25) -> (-3, 15.25) construction
  line L35 (-10.5, -30.75) -> (-4, -30.75) construction
  line L36 (-9.4847, -24.85) -> (-9.4847, -31.5493) construction
  line L37 (11, 32.75) -> (-11, 32.75)
  line L38 (-11, 32.75) -> (-11, 17.75)
  line L39 (-11, 17.75) -> (11, 17.75)
  line L40 (11, 17.75) -> (11, 32.75)
  line L41 (11, 32.75) -> (-11, 17.75) construction
  line L42 (-11, 32.75) -> (11, 17.75) construction
  line L43 (11, 17.75) -> (12.5, 17.75)
  line L44 (-11, 17.75) -> (-12.5, 17.75)
  line L45 (11, 17.75) -> (11, 16.6229)
  line L46 (-11, 17.75) -> (-11, 16.6227)
  point P0 (10.5, -30.75)
  point P1 (-10.5, -30.75)
  point P2 (-5, 13.25)
  point P3 (0, 25.25)
  point P4 (0, 32.75)
  point P5 (0, 32.75)
  dimension "d185" = 65.5
  dimension "d186" = 25
  dimension "d189" = 2
  dimension "d190" = 2
  dimension "d191" = 2
  dimension "d192" = 2
  dimension "d193" = 2
  dimension "d194" = 2
  dimension "d195" = 2
  dimension "d197" = 44
  dimension "d209" = 15
  dimension "d211" = 60
  dimension "d212" = 50
  dimension "d213" = 4
  dimension "d214" = 4
  dimension "d215" = 4
  dimension "d216" = 4
  dimension "d221" = 4
  dimension "d222" = 4
  dimension "d224" = 5.9
  dimension "d227" = 15
  dimension "d229" = 7.5
  dimension "d230" = 22
  constraint perpendicular L0 L1
  constraint parallel L0 L2
  constraint parallel L1 L3
  constraint horizontal L0
  constraint coincident L4 origin
  constraint coincident L5 origin
  constraint coincident P0 A0.centre
  constraint parallel L3 L6
  constraint perpendicular L3 L7
  constraint coincident L7 L8.start
  constraint coincident L1 L8.start
  constraint coincident L4 L9.end
  constraint perpendicular L7 L9
  constraint coincident L1 L10.end
  constraint midpoint L2 L12.start
  constraint perpendicular L0 L12
  constraint symmetric L8.start L12 L13.end
  constraint symmetric L8.end L12 L14.start
  constraint symmetric L9.end L12 L14.end
  constraint symmetric L10.end L12 L13.start
  constraint perpendicular L17 L18
  constraint parallel L17 L19
  constraint parallel L18 L20
  constraint horizontal L17
  constraint coincident L21 P0
  constraint coincident L22 P0
  constraint perpendicular L23 L24
  constraint parallel L23 L25
  constraint parallel L24 L26
  constraint horizontal L23
  constraint coincident L27 P1
  constraint coincident L28 P1
  constraint coincident P1 A1.centre
  constraint perpendicular L29 L30
  constraint parallel L29 L31
  constraint parallel L30 L32
  constraint horizontal L29
  constraint coincident L33 P2
  constraint coincident L34 P2
  constraint coincident P2 A2.centre
  constraint perpendicular L26 L35
  constraint vertical L36
  constraint perpendicular L37 L38
  constraint parallel L37 L39
  constraint parallel L38 L40
  constraint horizontal L37
  constraint coincident L41 P3
  constraint coincident L42 P3
  constraint coincident L12 P3
  constraint midpoint L0 P5
  constraint midpoint L37 P5
  constraint perpendicular L13 L43
  constraint perpendicular L39 L45
  constraint vertical L46
  measures "d185" distance of L0.end L1.end
  measures "d186" distance of L1.end L2.end
  measures "d189" diameter of A0
  measures "d190" diameter of A1
  measures "d191" diameter of A2
  measures "d192" distance of L3 P0
  measures "d193" distance of L2 P0
  measures "d194" distance of L2 P1
  measures "d195" distance of L1 P1
  measures "d197" vertical distance of P0 P2
  measures "d209" distance of L0 L7
  measures "d211" angle of L1 L8
  measures "d212" angle of L1 L10
  measures "d213" distance of L2.end L19.end
  measures "d214" distance of L17.end L2.end
  measures "d215" distance of L23.end L1.end
  measures "d216" distance of L1.end L25.end
  measures "d221" distance of L29.end L30.end
  measures "d222" distance of L30.end L31.end
  measures "d224" distance of L9.end L35
  measures "d227" distance of L37.end L38.end
  measures "d229" distance of P2 L11
  measures "d230" distance of L38 L40
extrude "Extrude1" add sketch "bed" along normal blind 3 separate body contours L0 L3 L40 L43 | L0 L37 L38 L39 L40 | L3 L13 L14 L15 L16 | L15 L43 L45 | L0 L1 L38 L44 | L1 L2 L3 L8 L9 L10 L14 L15 L16 L17 L20 L23 L26 L39 L45 L46 | L8 L44 L46 | L2 L3 L17 L18 L19 L20 | L1 L8 L9 L10 L11 | L1 L2 L23 L24 L25 L26 | A0 | A1 | A2 | L29 L30 L31 L32 makes body 3 in component "esp_bed"
extrude "Extrude2" cut sketch "bed" along normal up to surface (3 mm away) contours A0 | A1 | A2 bodies 3 in component "esp_bed"
extrude "Extrude3" cut sketch "bed" along normal up to surface (3 mm away) contours L3 L13 L14 L15 L16 | L1 L8 L9 L10 L11 bodies 3 in component "esp_bed"
extrude "Extrude4''" add sketch "bed" against normal blind 1.5 contours L2 L3 L17 L18 L19 L20 | L1 L2 L23 L24 L25 L26 bodies 3 in component "esp_bed"
extrude "Extrude5''" add sketch "bed" against normal blind 1.5 contours L29 L30 L31 L32 bodies 3 in component "esp_bed"
extrude "Extrude7'" cut sketch "bed" along normal up to surface (3 mm away) contours L0 L3 L40 L43 | L15 L43 L45 | L0 L1 L38 L44 | L8 L44 L46 bodies 3 in component "esp_bed"
sketch "number" plane through (0, 0, 0) normal (0, 1, 0) x (-1, 0, 0) in component "battery_cap"
  circle A0 centre (0, 0) radius 21.25
  line L0 (-9.5, -16) -> (-9.5, -3)
  line L1 (-9.5, -3) -> (9.5, -3)
  line L2 (9.5, -3) -> (9.5, -16)
  line L3 (9.5, -16) -> (-9.5, -16)
  line L4 (-5.5066, 18.4921) -> (-7.6219, 18.4921)
  line L5 (-7.6219, 18.4921) -> (-7.6219, 18.9989)
  line L6 (-7.6219, 18.9989) -> (-4.9383, 18.9989)
  line L7 (-4.9383, 18.9989) -> (-4.9383, 14.704)
  line L8 (-4.9383, 14.704) -> (-5.5066, 14.704)
  line L9 (-5.5066, 14.704) -> (-5.5066, 18.4921)
  line L10 (7.6067, 14.704) -> (7.0383, 14.704)
  line L11 (7.0383, 14.704) -> (7.0383, 18.9989)
  line L12 (7.0383, 18.9989) -> (7.6067, 18.9989)
  line L13 (7.6067, 18.9989) -> (7.6067, 14.704)
  line L14 (-3.3914, 14.704) -> (-3.9598, 14.704)
  line L15 (-3.9598, 14.704) -> (-3.9598, 18.9989)
  line L16 (-3.9598, 18.9989) -> (-3.3914, 18.9989)
  line L17 (-3.3914, 18.9989) -> (-3.3914, 14.704)
  spline S0 degree 3 poles (3.2854, 18.7118) (3.3618, 18.7564) (3.5231, 18.8505) (3.7033, 18.8998) (3.7981, 18.9257) knots 0 0 0 0 0.026441 0.055764 0.055764 0.055764 0.055764
  spline S1 degree 3 poles (3.7981, 18.9257) (3.9049, 18.947) (4.1321, 18.9924) (4.3638, 18.9966) (4.4865, 18.9989) knots 0 0 0 0 0.032619 0.069359 0.069359 0.069359 0.069359
  line L18 (4.4865, 18.9989) -> (6.0363, 18.9989)
  line L19 (6.0363, 18.9989) -> (6.0363, 14.704)
  line L20 (6.0363, 14.704) -> (4.5568, 14.704)
  spline S2 degree 3 poles (4.5568, 14.704) (4.4092, 14.7046) (4.1526, 14.7056) (3.8996, 14.7477) (3.7922, 14.7655) knots 0 0 0 0 0.044192 0.07682 0.07682 0.07682 0.07682
  spline S3 degree 3 poles (3.7922, 14.7655) (3.6749, 14.7985) (3.4461, 14.863) (3.2553, 15.0043) (3.1623, 15.0731) knots 0 0 0 0 0.036228 0.07062 0.07062 0.07062 0.07062
  spline S4 degree 3 poles (3.1623, 15.0731) (3.0557, 15.1769) (2.8384, 15.3885) (2.7172, 15.6667) (2.6555, 15.8085) knots 0 0 0 0 0.044179 0.090072 0.090072 0.090072 0.090072
  spline S5 degree 3 poles (2.6555, 15.8085) (2.6059, 15.9664) (2.5019, 16.2982) (2.4912, 16.6459) (2.4856, 16.828) knots 0 0 0 0 0.049425 0.103791 0.103791 0.103791 0.103791
  spline S6 degree 3 poles (2.4856, 16.828) (2.4892, 16.9826) (2.4961, 17.2759) (2.5665, 17.5606) (2.5998, 17.6952) knots 0 0 0 0 0.046231 0.087702 0.087702 0.087702 0.087702
  spline S7 degree 3 poles (2.5998, 17.6952) (2.6384, 17.8127) (2.711, 18.0336) (2.8348, 18.2302) (2.8928, 18.3221) knots 0 0 0 0 0.036947 0.069434 0.069434 0.069434 0.069434
  spline S8 degree 3 poles (2.8928, 18.3221) (2.9522, 18.3988) (3.0661, 18.5458) (3.2144, 18.658) (3.2854, 18.7118) knots 0 0 0 0 0.028941 0.055527 0.055527 0.055527 0.055527
  line L21 (-0.0691, 18.9989) -> (1.1731, 15.3426)
  line L22 (1.1731, 15.3426) -> (1.1731, 18.9989)
  line L23 (1.1731, 18.9989) -> (1.7209, 18.9989)
  line L24 (1.7209, 18.9989) -> (1.7209, 14.704)
  line L25 (1.7209, 14.704) -> (0.8654, 14.704)
  line L26 (0.8654, 14.704) -> (-0.1512, 17.745)
  spline S9 degree 3 poles (-0.1512, 17.745) (-0.1921, 17.8686) (-0.262, 18.0801) (-0.3286, 18.2925) (-0.3562, 18.3807) knots 0 0 0 0 0.039074 0.066801 0.066801 0.066801 0.066801
  spline S10 degree 3 poles (-0.3562, 18.3807) (-0.3872, 18.2842) (-0.4612, 18.054) (-0.5394, 17.8252) (-0.5848, 17.6923) knots 0 0 0 0 0.030412 0.072542 0.072542 0.072542 0.072542
  line L27 (-0.5848, 17.6923) -> (-1.6131, 14.704)
  line L28 (-1.6131, 14.704) -> (-2.3777, 14.704)
  line L29 (-2.3777, 14.704) -> (-2.3777, 18.9989)
  line L30 (-2.3777, 18.9989) -> (-1.8299, 18.9989)
  line L31 (-1.8299, 18.9989) -> (-1.8299, 15.4042)
  line L32 (-1.8299, 15.4042) -> (-0.5818, 18.9989)
  line L33 (-0.5818, 18.9989) -> (-0.0691, 18.9989)
  line L34 (15.5975, 10.0576) -> (-15.5627, 10.0576) construction
  line L35 (-15.5627, 10.0576) -> (-15.5627, -1.9424) construction
  line L36 (-15.5627, -1.9424) -> (15.5975, -1.9424) construction
  line L37 (15.5975, -1.9424) -> (15.5975, 10.0576) construction
  constraint perpendicular L34 L35
  constraint parallel L34 L36
  constraint parallel L35 L37
component "battery_cap" placed x (1, 0, 0) y (0, 1, 0) z (0, 0, 1) at (0, 0, 59)
component "esp_cap" placed x (1, 0, 0) y (0, 1, 0) z (0, 0, 1) at (0, 0, 0)
component "esp_bed" placed x (1, 0, 0) y (0, 1, 0) z (0, 0, 1) at (65, 0, 0)
equation "cap_thickness = 3.5 mm"
equation "cap_diameter = 42.5 mm"
equation "switch_length = 19 mm"
equation "switch_width = 13 mm"
equation "cap_ext_extrude = 15 mm"
equation "cap_int_extrude = 15 mm"
equation "battery_length = 42 mm"
equation "Battery_width = 33.5 mm"
equation "Battery_thickness = 6 mm"
equation "esp_bed_length = 65.5 mm"
equation "esp_bed_width = 25 mm"
equation "esp_bed_thickness = 3 mm"
equation "usb_length = 10 mm"
equation "usb_width = 5 mm"
equation "reset_length = 5 mm"
equation "reset_width = 7 mm"
equation "esp_bed_hole_diameter = 2 mm"
equation "button_thickness = 2 mm"
equation "button_length = 12.5 mm"
equation "button_diameter = 8 mm"
equation "d29 = cap_diameter"
equation "d30 = cap_thickness"
equation "d41 = -cap_thickness"
equation "d43 = cap_ext_extrude"
equation "d45 = -cap_thickness"
equation "d46 = cap_int_extrude"
equation "d48 = switch_length"
equation "d49 = switch_width"
equation "d51 = Battery_width * 0.7"
equation "d52 = Battery_thickness - 0.4 mm"
equation "battery_offset = 2 mm"
equation "d29_1 = cap_diameter"
equation "d30_1 = cap_thickness"
equation "d41_1 = -cap_thickness"
equation "d43_1 = cap_ext_extrude"
equation "d45_1 = -cap_thickness"
equation "d46_1 = cap_int_extrude + cap_thickness"
equation "d65 = esp_bed_width"
equation "d66 = esp_bed_thickness / 2"
equation "d70 = reset_length"
equation "d71 = reset_width"
equation "d74 = usb_length"
equation "d75 = usb_width"
equation "usb_offset = -2.5 mm"
equation "snap_thickness = 1 mm"
equation "snap_length = 3 mm"
equation "d108 = -cap_thickness + 1 mm"
equation "d111 = button_diameter"
equation "d113 = button_length"
equation "d114 = button_length"
equation "d117 = snap_thickness"
equation "d118 = snap_length"
equation "d119 = button_length / 2"
equation "snap_size = button_thickness - button_hole + 4 mm"
equation "button_hole = 1 mm"
equation "d155 = button_length"
equation "d156 = button_length"
equation "d159 = button_length / 2"
equation "d160 = button_length"
equation "d163 = -button_thickness"
equation "d168 = cap_thickness"
equation "d181 = battery_offset"
equation "d182 = battery_offset"
equation "d183 = cap_int_extrude"
equation "d185 = esp_bed_length"
equation "d186 = esp_bed_width"
equation "d187 = esp_bed_thickness"
equation "d189 = esp_bed_hole_diameter"
equation "d190 = esp_bed_hole_diameter"
equation "d191 = esp_bed_hole_diameter"
equation "d201 = d200"
equation "d202 = esp_bed_thickness + 0.25 mm"
equation "d203 = d202"
equation "d204 = esp_bed_thickness / 2"
equation "d205 = esp_bed_thickness / 2"
equation "d206 = d205"
equation "d207 = cap_int_extrude + cap_thickness"
equation "d209 = cap_int_extrude"
equation "d227 = cap_int_extrude"
